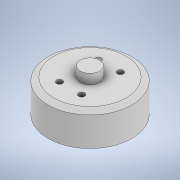
# Autodesk Inventor part: burshless_20_top
Saved by Autodesk Inventor 2020 (Build 240168000, 168)
## iProperties
Created: 2020-08-02
Part Number: burshless_20_top
Material: Generic
Document SubType Name: Modeling
Designer: psrobotics
Density: 1 g/cm^3
Appearance: Default
Author: psrobotics
Autodesk Inventor part; units mm, degrees
ref_plane "YZ Plane" through (0, 0, 0) normal (1, 0, 0) x (0, 1, 0)
ref_plane "XZ Plane" through (0, 0, 0) normal (0, 1, 0) x (-1, 0, 0)
ref_plane "XY Plane" through (0, 0, 0) normal (0, 0, 1) x (1, 0, 0)
sketch "Sketch1" plane through (0, 0, 0) normal (0, 1, 0) x (-1, 0, 0)
  circle A0 centre (0, 0) radius 11
  dimension "d0" = 22
  constraints: 1 centre point, 1 coincident
  measures "d0" diameter of A0
extrude "Extrusion1" add sketch "Sketch1" along normal blind 8.5
sketch "Sketch2" plane through (0, 8.5, 0) normal (0, 1, 0) x (1, 0, 0)
  circle A0 centre (0, 0) radius 2.5
  dimension "d3" = 5
  constraints: 1 centre point, 1 coincident
  measures "d3" diameter of A0
extrude "Extrusion2" add sketch "Sketch2" along normal blind 2.6
chamfer "Chamfer1" distance 1.5 angle 30 1 edges at (11, 8.5, 0) measured on face at (-8.0601, 8.5, -0.8775)
sketch "Sketch3" plane through (0, 0, 0) normal (0, -1, 0) x (1, 0, 0)
  circle A0 centre (0, 0) radius 10.25
  dimension "d9" = 20.5
  constraints: 1 centre point, 1 coincident
  measures "d9" diameter of A0
extrude "Extrusion3" cut sketch "Sketch3" against normal blind 7
sketch "Sketch4" plane through (0, 8.5, 0) normal (0, 1, 0) x (1, 0, 0)
  circle A0 centre (0, 0) radius 2.5 projected
  circle A1 centre (0, 0) radius 9.5 projected
  line L0 (-2.9, 5.1) -> (2.9, 5.1)
  line L1 (2.9, 5.1) -> (2.9, -5.1)
  line L2 (2.9, -5.1) -> (-2.9, -5.1)
  line L3 (-2.9, -5.1) -> (-2.9, 5.1)
  line L4 (-2.9, 5.1) -> (2.9, -5.1) construction
  line L5 (2.9, 5.1) -> (-2.9, -5.1) construction
  dimension "d12" = 5.8
  dimension "d13" = 10.2
  constraints: 12 end point, 2 midpoint, 2 parallel, 1 horizontal, 1 perpendicular
  measures "d12" distance of L0.start L0.end
  measures "d13" distance of L0.end L1.end
hole "Hole1" at (-2.9, 8.5, -5.1) at (2.9, 8.5, -5.1) at (-2.9, 8.5, 5.1) at (2.9, 8.5, 5.1) direction (0, -1, 0) diameter 1.6 depth 17
sketch "Sketch5" plane through (0, 0, 0) normal (0, -1, 0) x (1, 0, 0)
  circle A0 centre (-2.9, 5.1) radius 0.8 projected
  circle A1 centre (-2.9, -5.1) radius 0.8 projected
  circle A2 centre (2.9, -5.1) radius 0.8 projected
  circle A3 centre (2.9, 5.1) radius 0.8 projected
  circle A4 centre (0, 0) radius 10.25 projected
  circle A5 centre (0, 0) radius 10.25 projected
  circle A6 centre (0, 0) radius 11 projected
  line L0 (-10.5, -1.4) -> (-10, -1.4)
  line L1 (-10, -1.4) -> (-10, 1.4)
  line L2 (-10, 1.4) -> (-10.5, 1.4)
  line L3 (-10.5, 1.4) -> (-10.5, -1.4)
  line L4 (-10.5, -1.4) -> (-10, 1.4) construction
  line L5 (-10, -1.4) -> (-10.5, 1.4) construction
  line L6 (0, 0) -> (-10.25, 0)
  dimension "d21" = 0.5
  dimension "d22" = 2.8
  constraints: 14 end point, 2 horizontal, 2 midpoint, 2 parallel, 1 horizontal alignment, 1 perpendicular, 1 other
  measures "d21" distance of L0.start L0.end
  measures "d22" distance of L1.end L0.end
extrude "Extrusion4" add sketch "Sketch5" against normal blind 7 contours L2 L1 L6 A4 | A4 L0 L3 L2 | A4 L6 L1 L0
pattern_circular "Circular Pattern1" count 18 over 360 about axis through (0, 0, 0) along (0, 1, 0) of "Extrusion4"
body "Solid1"
